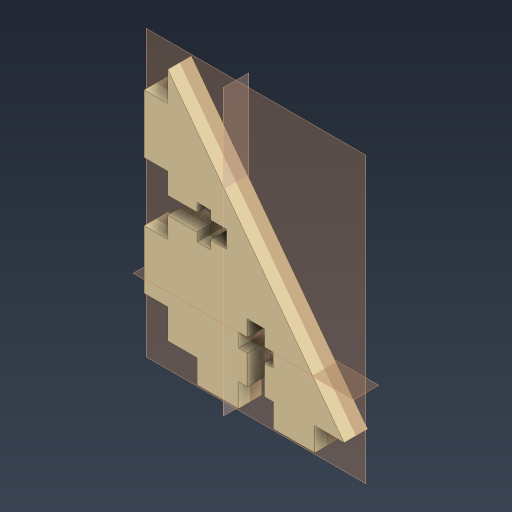
# Autodesk Inventor part: Рёбра_жёсткости
Saved by Autodesk Inventor 2023.2 (Build 272271030, 271C)
## iProperties
Created: 2025-12-29
Part Number: Рёбра_жёсткости
Material: Типовые
Document SubType Name: Modeling
Designer: Олег Коноваленко
Density: 1 g/cm^3
Appearance: Пшеничный
Author: Олег Коноваленко
Autodesk Inventor part; units mm, degrees
sketch "Эскиз1" plane through (0, 0, 0) normal (0, 0, 1) x (1, 0, 0)
  line L0 (-9.6, 32.8) -> (-9.6, -7.2)
  line L1 (-9.6, -7.2) -> (20.4, -7.2)
  line L2 (20.4, -7.2) -> (-9.6, 32.8)
  line L3 (-9.6, -7.2) -> (9.6, 7.2) construction
  line L4 (-4.6, -7.2) -> (2.4, -7.2)
  line L5 (2.4, -7.2) -> (2.4, -11.2)
  line L6 (2.4, -11.2) -> (-4.6, -11.2)
  line L7 (-4.6, -11.2) -> (-4.6, -7.2)
  line L8 (8.4, -7.2) -> (15.4, -7.2)
  line L9 (15.4, -7.2) -> (15.4, -11.2)
  line L10 (15.4, -11.2) -> (8.4, -11.2)
  line L11 (8.4, -11.2) -> (8.4, -7.2)
  line L12 (-9.6, 27.8) -> (-13.6, 27.8)
  line L13 (-13.6, 27.8) -> (-13.6, 17.8)
  line L14 (-13.6, 17.8) -> (-9.6, 17.8)
  line L15 (-9.6, 17.8) -> (-9.6, 27.8)
  line L16 (-9.6, -2.2) -> (-13.6, -2.2)
  line L17 (-13.6, -2.2) -> (-13.6, 7.8)
  line L18 (-13.6, 7.8) -> (-9.6, 7.8)
  line L19 (-9.6, 7.8) -> (-9.6, -2.2)
  point P0 (0, 0)
  point P1 (0, 0)
  point P2 (-9.6, 17.8)
  point P3 (-9.6, 7.8)
  dimension "d0" = 30
  dimension "d1" = 40
  dimension "d2" = 10
  dimension "d3" = 5
  dimension "d4" = 4
  dimension "d5" = 5
  dimension "d6" = 5
  dimension "d7" = 7
  dimension "d8" = 5
  constraints: 40 end point, 8 parallel, 6 perpendicular, 5 equal length, 5 point on line, 4 horizontal, 1 coincident, 1 midpoint, 1 vertical
  measures "d0" distance of L0.end L1.end
  measures "d1" distance of L0.start L0.end
  measures "d2" distance of L12.end L13.end
  measures "d3" distance from line of L0.start L12
  measures "d4" distance of L13.end L14.end
  measures "d5" distance from line of L0.end L16
  measures "d6" distance from line of L0.end L7
  measures "d7" distance of L5.end L6.end
  measures "d8" distance from line of L1.end L9
extrude "Выдавливание1" add sketch "Эскиз1" along normal mid plane 4
sketch "Эскиз2" plane through (0, 0, 2) normal (0, 0, 1) x (1, 0, 0)
  line L0 (-9.6, 17.8) -> (-9.6, 7.8) projected
  line L1 (-9.6, 14.25) -> (0.4, 14.25)
  line L2 (0.4, 14.25) -> (0.4, 11.35)
  line L3 (0.4, 11.35) -> (-9.6, 11.35)
  line L4 (-9.6, 11.35) -> (-9.6, 14.25)
  line L5 (2.4, -7.2) -> (8.4, -7.2) projected
  line L6 (3.95, -7.2) -> (6.85, -7.2)
  line L7 (6.85, -7.2) -> (6.85, 2.8)
  line L8 (6.85, 2.8) -> (3.95, 2.8)
  line L9 (3.95, 2.8) -> (3.95, -7.2)
  line L10 (-4.6, 15.7) -> (-2.3, 15.7)
  line L11 (-2.3, 15.7) -> (-2.3, 9.9)
  line L12 (-2.3, 9.9) -> (-4.6, 9.9)
  line L13 (-4.6, 9.9) -> (-4.6, 15.7)
  line L14 (2.5, 0.1) -> (8.3, 0.1)
  line L15 (8.3, 0.1) -> (8.3, -2.2)
  line L16 (8.3, -2.2) -> (2.5, -2.2)
  line L17 (2.5, -2.2) -> (2.5, 0.1)
  line L18 (-9.6, 12.8) -> (0.4, 12.8) construction
  line L19 (5.4, 2.8) -> (5.4, -7.2) construction
  point P0 (0, 0)
  point P1 (-2.3, 12.8)
  point P2 (5.4, 0.1)
  point P3 (-4.6, 14.25)
  point P4 (-4.6, 11.35)
  point P5 (-2.3, 11.35)
  point P6 (-2.3, 14.25)
  point P7 (3.95, -2.2)
  point P8 (6.85, -2.2)
  point P9 (6.85, 0.1)
  point P10 (3.95, 0.1)
  dimension "d11" = 2.9
  dimension "d12" = 10
  dimension "d13" = 2.3
  dimension "d14" = 5.8
  dimension "d15" = 5
  dimension "d16" = 5
  constraints: 36 end point, 8 midpoint, 8 parallel, 8 perpendicular, 4 horizontal, 4 point on line, 1 vertical
  measures "d11" distance of L1.end L2.end
  measures "d12" distance of L2.end L3.end
  measures "d13" distance of L10.start L10.end
  measures "d14" distance of L10.end L11.end
  measures "d15" distance between parallel lines of L0 L13
  measures "d16" distance between parallel lines of L5 L16
extrude "Выдавливание2" cut sketch "Эскиз2" against normal up to next
